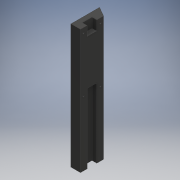
# Autodesk Inventor part: HB01
Saved by Autodesk Inventor 2017 (Build 210142000, 142)
## iProperties
Created: 2019-05-20
Part Number: HB01
Material: Polyethylene, High Density
Document SubType Name: Modeling
Designer: Dell
Density: 0.952 g/cm^3
Appearance: Smooth - Black
Mass: 478.234 g
Surface Area: 750.07 cm^2
Volume: 502.346 cm^3
Author: Dell
Autodesk Inventor part; units mm, degrees
ref_plane "YZ Plane" through (0, 0, 0) normal (1, 0, 0) x (0, 1, 0)
ref_plane "XZ Plane" through (0, 0, 0) normal (0, 1, 0) x (-1, 0, 0)
ref_plane "XY Plane" through (0, 0, 0) normal (0, 0, 1) x (1, 0, 0)
sketch "Sketch1" plane through (0, 0, 0) normal (0, 0, 1) x (1, 0, 0)
  line L0 (0, 0) -> (0, 76.2)
  line L1 (0, 76.2) -> (25.4, 61.5353)
  line L2 (25.4, 61.5353) -> (25.4, 0)
  line L3 (25.4, 0) -> (0, 0)
  dimension "d0" = 25.4
  dimension "d1" = 76.2
  dimension "d2" = 60
  constraints: 8 end point, 1 parallel, 1 perpendicular, 1 vertical
  measures "d0" distance between parallel lines of L2 L0
  measures "d1" distance of L0.start L0.end
  measures "d2" angle of L0 L1
extrude "Extrusion1" add sketch "Sketch1" along normal blind 330.2
sketch "Sketch3" plane through (0, 0, 330.2) normal (0, 0, 1) x (1, 0, 0)
  line L0 (12.7, 43.4677) -> (25.4, 43.4677)
  line L1 (25.4, 43.4677) -> (25.4, 18.0677)
  line L2 (25.4, 18.0677) -> (12.7, 18.0677)
  line L3 (12.7, 18.0677) -> (12.7, 43.4677)
  line L4 (25.4, 0) -> (25.4, 61.5353) projected
  point P0 (0, 0)
  point P1 (25.4, 30.7677)
  dimension "d5" = 12.7
  dimension "d6" = 25.4
  constraints: 8 end point, 2 midpoint, 2 parallel, 1 horizontal, 1 perpendicular, 1 point on line
  measures "d5" distance of L1.end L2.end
  measures "d6" distance of L0.end L1.end
extrude "Extrusion2" cut sketch "Sketch3" against normal blind 185
sketch "Sketch4" plane through (0, 0, 0) normal (0, 0, -1) x (-1, 0, 0)
  line L0 (-12.7, 18.0677) -> (-12.7, 43.4677) projected
  line L1 (-12.7, 18.0677) -> (-12.7, 43.4677) projected
  line L2 (-25.4, 18.0677) -> (-12.7, 18.0677) projected
  line L3 (-25.4, 43.4677) -> (-25.4, 18.0677) projected
  line L4 (-12.7, 43.4677) -> (-25.4, 43.4677) projected
  point P0 (0, 0)
extrude "Extrusion3" cut sketch "Sketch4" against normal blind 25.4
ref_plane "Work Plane1" through (0, 0, 165.1) normal (0, 0, 1) x (1, 0, 0)
mirror "Mirror1" about plane through (0, 0, 165.1) normal (0, 0, 1) of "Extrusion1", "Extrusion2", "Extrusion3"
sketch "Sketch5" plane through (25.4, 61.5353, 330.2) normal (1, 0, 0) x (0, 0, -1)
  circle A0 centre (12.7, -8) radius 2
  circle A1 centre (12.7, -53.5353) radius 2
  line L0 (25.4, -18.0677) -> (25.4, -43.4677) projected
  line L1 (330.2, 0) -> (0, 0) projected
  line L2 (330.2, -61.5353) -> (0, -61.5353) projected
  circle A2 centre (157.9, -8) radius 2
  circle A3 centre (157.9, -53.5353) radius 2
  line L3 (145.2, -43.4677) -> (145.2, -18.0677) projected
  dimension "d11" = 4
  dimension "d12" = 4
  dimension "d13" = 12.7
  dimension "d14" = 8
  dimension "d15" = 8
  dimension "d16" = 4
  dimension "d17" = 4
  dimension "d18" = 12.7
  constraints: 4 centre point, 2 horizontal alignment, 2 vertical alignment
  measures "d11" diameter of A0
  measures "d12" diameter of A1
  measures "d13" distance from line of A0.centre L0
  measures "d14" distance from line of L1 A0.centre
  measures "d15" distance from line of L2 A1.centre
  measures "d16" diameter of A2
  measures "d17" diameter of A3
  measures "d18" distance from line of L3 A2.centre
extrude "Extrusion4" cut sketch "Sketch5" against normal through all
sketch "Sketch6" plane through (0, 0, 0) normal (-1, 0, 0) x (0, 0, 1)
  circle A0 centre (317.5, 53.5353) radius 2 projected
  circle A1 centre (317.5, 8) radius 2 projected
  circle A2 centre (172.3, 8) radius 2 projected
  circle A3 centre (172.3, 53.5353) radius 2 projected
  circle A4 centre (317.5, 53.5353) radius 2 projected
  circle A5 centre (317.5, 53.5353) radius 6.5
  circle A6 centre (317.5, 8) radius 2 projected
  circle A7 centre (317.5, 8) radius 6.5
  circle A8 centre (172.3, 8) radius 6.5
  circle A9 centre (172.3, 53.5353) radius 6.5
  point P0 (0, 0)
  dimension "d21" = 13
  dimension "d22" = 13
  dimension "d23" = 13
  dimension "d24" = 13
  constraints: 4 centre point, 4 coincident
  measures "d21" diameter of A5
  measures "d22" diameter of A7
  measures "d23" diameter of A8
  measures "d24" diameter of A9
extrude "Extrusion5" cut sketch "Sketch6" against normal blind 12.7 contours A0 | A1 | A2 | A3 | A5 | A7 | A8 | A9
sketch "Sketch8" plane through (0, 0, 0) normal (0, 0, -1) x (-1, 0, 0)
  line L0 (-12.7, 13.1) -> (-12.7, 63.1)
  line L1 (-25.4, 0) -> (0, 0) projected
  line L2 (0, 0) -> (0, 76.2) projected
  circle A0 centre (-12.7, 13.1) radius 2
  circle A1 centre (-12.7, 63.1) radius 2
  point P0 (-12.7, 0)
  point P1 (-12.7, 38.1)
  point P2 (0, 38.1)
  dimension "d32" = 50
  dimension "d33" = 4
  dimension "d34" = 4
  constraints: 3 midpoint, 2 centre point, 2 coincident, 2 end point, 1 horizontal alignment, 1 vertical, 1 vertical alignment
  measures "d32" distance of L0.start L0.end
  measures "d33" diameter of A0
  measures "d34" diameter of A1
extrude "Extrusion7" cut sketch "Sketch8" against normal blind 38.1
body "Solid1"
